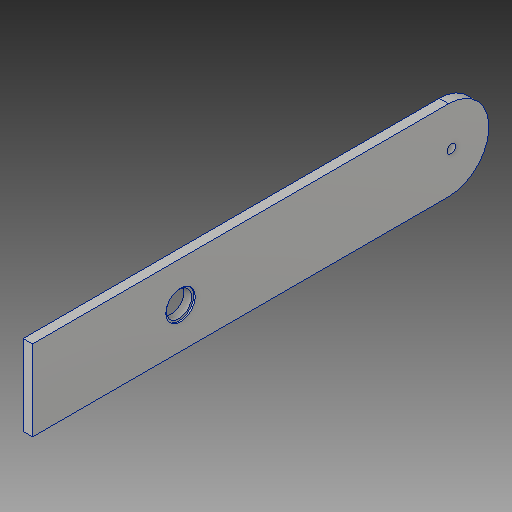
# Autodesk Inventor part: Outer Plate Module
Saved by Autodesk Inventor 2019.4 (Build 234330000, 330)
## iProperties
Created: 2020-01-01
Part Number: Outer Plate Module
Material: Aluminum 6061
Document SubType Name: Modeling
Designer: Mark
Mass: 241.565 g
Surface Area: 300.18 cm^2
Volume: 89.4685 cm^3
Density: 2.7 g/cm^3
Appearance: Aluminum - Flat
Author: Mark
Autodesk Inventor part; units mm, degrees
ref_plane "YZ Plane" through (0, 0, 0) normal (1, 0, 0) x (0, 1, 0)
ref_plane "XZ Plane" through (0, 0, 0) normal (0, 1, 0) x (-1, 0, 0)
ref_plane "XY Plane" through (0, 0, 0) normal (0, 0, 1) x (1, 0, 0)
sketch "Sketch1" plane through (0, 0, 0) normal (1, 0, 0) x (0, 1, 0)
  circle A0 centre (0, 0) radius 9.5
  line L0 (-30, -110.28) -> (30, -110.28)
  line L1 (30, -110.28) -> (30, 110.28)
  line L2 (30, 110.28) -> (-30, 110.28)
  line L3 (-30, 110.28) -> (-30, -110.28)
  line L4 (-30, -110.28) -> (30, 110.28) construction
  line L5 (30, -110.28) -> (-30, 110.28) construction
  line L6 (30, -110.28) -> (-30, -110.28)
  line L7 (-30, -110.28) -> (-30, -229.72)
  line L8 (-30, -229.72) -> (30, -229.72)
  line L9 (30, -229.72) -> (30, -110.28)
  circle A1 centre (0, -201.7) radius 3.25
  dimension "d0" = 19
  dimension "d1" = 60
  dimension "d2" = 220.56
  dimension "d5" = 60
  dimension "d6" = 119.44
  dimension "d8" = 6.5
  dimension "d9" = 28.02
  dimension "d10" = 30
  constraints: 20 end point, 4 parallel, 2 centre point, 2 horizontal, 2 midpoint, 2 perpendicular, 1 coincident
  measures "d0" diameter of A0
  measures "d1" distance of L2.end L1.end
  measures "d2" distance of L1.end L0.end
  measures "d5" distance of L8.end L7.end
  measures "d6" distance of L7.end L6.end
  measures "d8" diameter of A1
  measures "d9" distance from line of L8 A1.centre
  measures "d10" distance from line of L7 A1.centre
extrude "Extrusion1" add sketch "Sketch1" along normal blind 7
fillet "Fillet1" radius 30 2 edges at (3.5, -30, -229.72) (3.5, 30, -229.72)
sketch "Sketch2" plane through (7, 0, 0) normal (-1, 0, 0) x (0, 0, 1)
  circle A0 centre (0, 0) radius 11
  dimension "d11" = 22
  constraints: 1 centre point, 1 coincident
  measures "d11" diameter of A0
extrude "Extrusion2" cut sketch "Sketch2" along normal blind 1.2
body "Solid1"
